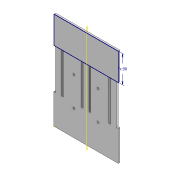
# Autodesk Inventor part: deepest_layer
Saved by Autodesk Inventor 2020 (Build 240168000, 168)
## iProperties
Created: 2021-05-08
Part Number: deepest_layer
Material: Generic
Document SubType Name: Modeling
Designer: Hsu Daniel
Density: 1 g/cm^3
Appearance: Default
Author: Hsu Daniel
Autodesk Inventor part; units mm, degrees
ref_plane "YZ Plane" through (0, 0, 0) normal (1, 0, 0) x (0, 1, 0)
ref_plane "XZ Plane" through (0, 0, 0) normal (0, 1, 0) x (-1, 0, 0)
ref_plane "XY Plane" through (0, 0, 0) normal (0, 0, 1) x (1, 0, 0)
sketch "Sketch1" plane through (0, 0, 0) normal (0, 0, 1) x (1, 0, 0)
  line L0 (0, 0) -> (106.5, 0)
  line L1 (106.5, 0) -> (106.5, 232.6) construction
  line L2 (106.5, 232.6) -> (0, 232.6)
  line L3 (0, 232.6) -> (0, 0)
  line L4 (213, 0) -> (106.5, 0)
  line L5 (106.5, 232.6) -> (213, 232.6)
  line L6 (213, 232.6) -> (213, 0)
  line L7 (5.5, 100) -> (5.5, 232.599)
  line L8 (5.5, 232.599) -> (0, 232.599)
  line L9 (0, 232.599) -> (0, 100)
  line L10 (0, 100) -> (5.5, 100)
  line L11 (5.5, 100) -> (0, 232.599) construction
  line L12 (5.5, 232.599) -> (0, 100) construction
  line L13 (31, 100) -> (31, 232.599)
  line L14 (31, 232.599) -> (25.5, 232.599)
  line L15 (25.5, 232.599) -> (25.5, 100)
  line L16 (25.5, 100) -> (31, 100)
  line L17 (31, 100) -> (25.5, 232.599) construction
  line L18 (31, 232.599) -> (25.5, 100) construction
  line L19 (96.5, 100) -> (96.5, 232.599)
  line L20 (96.5, 232.599) -> (91.5, 232.599)
  line L21 (91.5, 232.599) -> (91.5, 100)
  line L22 (91.5, 100) -> (96.5, 100)
  line L23 (96.5, 100) -> (91.5, 232.599) construction
  line L24 (96.5, 232.599) -> (91.5, 100) construction
  line L25 (207.5, 100) -> (207.5, 232.599)
  line L26 (207.5, 232.599) -> (213, 232.599)
  line L27 (213, 232.599) -> (213, 100)
  line L28 (213, 100) -> (207.5, 100)
  line L29 (207.5, 100) -> (213, 232.599) construction
  line L30 (207.5, 232.599) -> (213, 100) construction
  line L31 (182, 100) -> (182, 232.599)
  line L32 (182, 232.599) -> (187.5, 232.599)
  line L33 (187.5, 232.599) -> (187.5, 100)
  line L34 (187.5, 100) -> (182, 100)
  line L35 (182, 100) -> (187.5, 232.599) construction
  line L36 (182, 232.599) -> (187.5, 100) construction
  line L37 (116.5, 100) -> (116.5, 232.599)
  line L38 (116.5, 232.599) -> (121.5, 232.599)
  line L39 (121.5, 232.599) -> (121.5, 100)
  line L40 (121.5, 100) -> (116.5, 100)
  line L41 (116.5, 100) -> (121.5, 232.599) construction
  line L42 (116.5, 232.599) -> (121.5, 100) construction
  line L43 (2.75, 166.2995) -> (94, 166.2995) construction
  point P0 (28.25, 166.2995)
  point P1 (210.25, 166.2995)
  point P2 (184.75, 166.2995)
  point P3 (119, 166.2995)
  point P4 (0, 100)
  point P5 (213, 100)
  point P6 (0, 232.599)
  dimension "d0" = 232.6
  dimension "d1" = 106.5
  dimension "d4" = 5.5
  dimension "d6" = 5.5
  dimension "d8" = 5
  dimension "d10" = 10
  dimension "d11" = 20
  dimension "d12" = 0
  dimension "d19" = 100
  dimension "d20" = 0.001
  constraints: 88 end point, 17 symmetric about line, 12 midpoint, 8 parallel, 4 perpendicular, 3 collinear, 2 horizontal
  measures "d0" distance of L1.end L0.end
  measures "d1" distance of L1.end L2.end
  measures "d4" distance of L8.end L7.end
  measures "d6" distance of L14.end L13.end
  measures "d8" distance of L20.end L19.end
  measures "d10" distance between parallel lines of L1 L19
  measures "d11" distance between parallel lines of L15 L7
  measures "d12" distance between parallel lines of L3 L9
  measures "d19" distance between parallel lines of L0 L16
  measures "d20" distance between parallel lines of L2 L8
extrude "Extrusion1" add sketch "Sketch1" along normal blind 5.5 contours L3 L10 L7 L2 L15 L16 L13 L21 L22 L19 L5 L37 L40 L39 L31 L34 L33 L25 L28 L6 L4 L0
ref_plane "Work Plane3" through (61.25, 100, 0) normal (1, 0, 0) x (0, 0, -1)
sketch "Sketch2" plane through (0, 0, 5.5) normal (0, 0, 1) x (1, 0, 0)
  line L0 (0, 232.6) -> (213, 232.6)
  line L1 (213, 232.6) -> (213, 322.6)
  line L2 (213, 322.6) -> (0, 322.6)
  line L3 (0, 322.6) -> (0, 232.6)
  line L4 (213, 232.599) -> (213, 232.6) projected
  point P0 (0, 0)
  dimension "d15" = 90
  constraints: 8 end point, 2 parallel, 1 coincident, 1 collinear, 1 horizontal, 1 perpendicular
  measures "d15" distance of L0.end L1.end
extrude "Extrusion2" add sketch "Sketch2" against normal blind 5.5
sketch "Sketch3" plane through (0, 0, 5.5) normal (0, 0, 1) x (1, 0, 0)
  line L0 (213, 322.6) -> (0, 322.6) construction
  line L1 (31, 232.599) -> (31, 100) construction
  line L2 (91.5, 100) -> (91.5, 232.599) construction
  line L3 (121.5, 232.599) -> (121.5, 100) construction
  line L4 (31, 166.2995) -> (91.5, 166.2995) construction
  line L5 (91.5, 166.2995) -> (121.5, 166.2995) construction
  line L6 (106.5, 166.2995) -> (106.5, 322.6) construction
  circle A0 centre (66.5, 182) radius 3.25
  circle A1 centre (66.5, 85) radius 3.25
  circle A2 centre (146.5, 182) radius 3.25
  circle A3 centre (146.5, 85) radius 3.25
  line L7 (66.5, 85) -> (66.5, 182) construction
  line L8 (0, 0) -> (213, 0) projected
  dimension "d21" = 6.5
  dimension "d23" = 97
  dimension "d28" = 40
  dimension "d29" = 85
  constraints: 8 end point, 5 midpoint, 4 centre point, 2 symmetric about line, 1 equal radius, 1 vertical, 2 other
  measures "d21" diameter of A0
  measures "d23" distance of L7.start L7.end
  measures "d28" distance between parallel lines of L6 L7
  measures "d29" distance from line of L7.start L8
extrude "Extrusion3" cut sketch "Sketch3" against normal blind 10
ref_plane "Work Plane4" through (106.5, 100, 0) normal (1, 0, 0) x (0, 0, -1)
equation "\"d0\" = sidewallL + Uthick"
equation "\"d10\" = 0.5 * midbottomw"
equation "\"d11\" = lrbottomw"
equation "\"d19\" = Uthick"
equation "\"d15\" = wireL"
equation "\"d28\" = 0.5 * marshdistance"
equation "\"thick\" = 0.5"
equation "\"lrlr\" = 19"
equation "\"lrmid\" = 19.9"
equation "\"lrdepth\" = 3.3"
equation "\"mlr\" = 16.6"
equation "\"mmid\" = 24.7"
equation "\"mdepth\" = 4.5"
equation "\"lrltotal\" = 126.6"
equation "\"mltotal\" = 126.6"
equation "\"lrbetween\" = 52.1"
equation "\"mbetween\" = 49.5"
equation "\"toler\" = 1"
equation "\"lrbottomw\" = 20"
equation "\"tight\" = 0.08"
equation "\"stuckw\" = 6"
equation "\"sidewallL\" = 132.6"
equation "\"heaterH\" = 117.3"
equation "\"Uthick\" = 100"
equation "\"stickL\" = 3.5"
equation "\"wireH\" = 25"
equation "\"wireL\" = 90"
equation "\"midbottomw\" = 20"
equation "\"marshdistance\" = 80"
body "Solid1"
